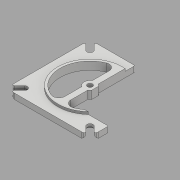
# Autodesk Inventor part: V4 In wall
Saved by Autodesk Inventor 2018 (Build 220112000, 112)
## iProperties
Created: 2020-01-08
Part Number: V4 In wall
Material: Generic
Document SubType Name: Modeling
Designer: user
Density: 1 g/cm^3
Appearance: Default
Author: user
Autodesk Inventor part; units mm, degrees
ref_plane "YZ Plane" through (0, 0, 0) normal (1, 0, 0) x (0, 1, 0)
ref_plane "XZ Plane" through (0, 0, 0) normal (0, 1, 0) x (-1, 0, 0)
ref_plane "XY Plane" through (0, 0, 0) normal (0, 0, 1) x (1, 0, 0)
sketch "Sketch1" plane through (0, 0, 0) normal (0, 0, 1) x (1, 0, 0)
  line L0 (-28.2, -35.2) -> (28.2, -35.2)
  line L1 (35.2, -28.2) -> (35.2, 28.2)
  line L2 (28.2, 35.2) -> (-28.2, 35.2)
  line L3 (-35.2, 28.2) -> (-35.2, -28.2)
  line L4 (-35.2, -35.2) -> (35.2, 35.2) construction
  line L5 (35.2, -35.2) -> (-35.2, 35.2) construction
  arc A0 (-28.2, 35.2) -> (-35.2, 28.2) centre (-28.2, 28.2) ccw
  arc A1 (35.2, 28.2) -> (28.2, 35.2) centre (28.2, 28.2) ccw
  arc A2 (-35.2, -28.2) -> (-28.2, -35.2) centre (-28.2, -28.2) ccw
  arc A3 (28.2, -35.2) -> (35.2, -28.2) centre (28.2, -28.2) ccw
  line L6 (-2.5, -24.8747) -> (2.5, -24.8747) construction
  line L7 (2.5, 24.8747) -> (-2.5, 24.8747) construction
  line L8 (-2.5, -24.8747) -> (2.5, 24.8747) construction
  line L9 (2.5, -24.8747) -> (-2.5, 24.8747) construction
  arc A4 (-9.375, 23.1756) -> (-9.375, -23.1756) centre (0, 0) ccw
  arc A5 (9.375, -23.1756) -> (9.375, 23.1756) centre (0, 0) ccw
  arc A6 (-2.5, 18.5405) -> (-9.375, 23.1756) centre (-7.5, 18.5405) ccw
  arc A7 (9.375, 23.1756) -> (2.5, 18.5405) centre (7.5, 18.5405) ccw
  arc A8 (-9.375, -23.1756) -> (-2.5, -18.5405) centre (-7.5, -18.5405) ccw
  arc A9 (2.5, -18.5405) -> (9.375, -23.1756) centre (7.5, -18.5405) ccw
  line L10 (2.5, 4.3301) -> (2.5, 18.5405)
  line L11 (-2.5, 18.5405) -> (-2.5, 4.3301)
  line L12 (-2.5, -4.3301) -> (-2.5, -18.5405)
  line L13 (2.5, -18.5405) -> (2.5, -4.3301)
  arc A10 (-2.5, 4.3301) -> (-2.5, -4.3301) centre (0, 0) ccw
  arc A11 (2.5, -4.3301) -> (2.5, 4.3301) centre (0, 0) ccw
  dimension "d0" = 70.4
  dimension "d1" = 7
  dimension "d3" = 5
  dimension "d4" = 25
  dimension "d5" = 5
  dimension "d7" = 5
  constraints: 28 end point, 28 point on circle, 20 tangent, 12 centre point, 10 point on line, 7 equal radius, 7 parallel, 4 midpoint, 4 perpendicular, 2 coincident, 2 horizontal
  measures "d0" distance of L4.end L5.end
  measures "d1" radius of A0
  measures "d3" distance of L7.end L7.start
  measures "d4" radius of A5
  measures "d5" radius of A6
  measures "d7" radius of A11
extrude "Extrusion1" add sketch "Sketch1" along normal blind 4.7
sketch "Sketch2" plane through (0, 0, 4.7) normal (0, 0, 1) x (1, 0, 0)
  circle A0 centre (0, 0) radius 27
  arc A1 (9.375, -23.1756) -> (9.375, 23.1756) centre (0, 0) ccw projected
  arc A2 (2.5, -18.5405) -> (9.375, -23.1756) centre (7.5, -18.5405) ccw projected
  line L0 (2.5, -18.5405) -> (2.5, -4.3301) projected
  arc A3 (2.5, -4.3301) -> (2.5, 4.3301) centre (0, 0) ccw projected
  line L1 (2.5, 4.3301) -> (2.5, 18.5405) projected
  arc A4 (9.375, 23.1756) -> (2.5, 18.5405) centre (7.5, 18.5405) ccw projected
  line L2 (-2.5, 18.5405) -> (-2.5, 4.3301) projected
  arc A5 (-2.5, 4.3301) -> (-2.5, -4.3301) centre (0, 0) ccw projected
  line L3 (-2.5, -4.3301) -> (-2.5, -18.5405) projected
  arc A6 (-9.375, -23.1756) -> (-2.5, -18.5405) centre (-7.5, -18.5405) ccw projected
  arc A7 (-9.375, 23.1756) -> (-9.375, -23.1756) centre (0, 0) ccw projected
  arc A8 (-2.5, 18.5405) -> (-9.375, 23.1756) centre (-7.5, 18.5405) ccw projected
  line L4 (28.2, 35.2) -> (-28.2, 35.2) projected
  arc A9 (-28.2, 35.2) -> (-35.2, 28.2) centre (-28.2, 28.2) ccw projected
  line L5 (-35.2, 28.2) -> (-35.2, -28.2) projected
  arc A10 (-35.2, -28.2) -> (-28.2, -35.2) centre (-28.2, -28.2) ccw projected
  line L6 (-28.2, -35.2) -> (28.2, -35.2) projected
  arc A11 (28.2, -35.2) -> (35.2, -28.2) centre (28.2, -28.2) ccw projected
  line L7 (35.2, -28.2) -> (35.2, 28.2) projected
  arc A12 (35.2, 28.2) -> (28.2, 35.2) centre (28.2, 28.2) ccw projected
  dimension "d10" = 54
  constraints: 1 centre point, 1 coincident
  measures "d10" diameter of A0
extrude "Extrusion2" add sketch "Sketch2" along normal blind 2 contours A0
sketch "Sketch3" plane through (0, 0, 0) normal (0, 0, -1) x (-1, 0, 0)
  line L0 (-27.5, -27.5) -> (27.5, -27.5) construction
  line L1 (27.5, -27.5) -> (27.5, 27.5) construction
  line L2 (27.5, 27.5) -> (-27.5, 27.5) construction
  line L3 (-27.5, 27.5) -> (-27.5, -27.5) construction
  line L4 (-27.5, -27.5) -> (27.5, 27.5) construction
  line L5 (27.5, -27.5) -> (-27.5, 27.5) construction
  line L6 (27.5, 27.5) -> (32.8233, 32.8233) construction
  line L7 (29.2678, 25.7322) -> (34.5911, 31.0555)
  line L8 (31.0555, 34.5911) -> (25.7322, 29.2678)
  arc A0 (25.7322, 29.2678) -> (29.2678, 25.7322) centre (27.5, 27.5) ccw
  arc A1 (34.5911, 31.0555) -> (31.0555, 34.5911) centre (32.8233, 32.8233) ccw
  arc A2 (35.2, 28.2) -> (28.2, 35.2) centre (28.2, 28.2) ccw construction
  line L9 (-25.7322, 29.2678) -> (-31.0555, 34.5911)
  arc A3 (-29.2678, 25.7322) -> (-25.7322, 29.2678) centre (-27.5, 27.5) ccw
  line L10 (-34.5911, 31.0555) -> (-29.2678, 25.7322)
  arc A4 (-31.0555, 34.5911) -> (-34.5911, 31.0555) centre (-32.8233, 32.8233) ccw
  line L11 (-29.2678, -25.7322) -> (-34.5911, -31.0555)
  arc A5 (-25.7322, -29.2678) -> (-29.2678, -25.7322) centre (-27.5, -27.5) ccw
  line L12 (-31.0555, -34.5911) -> (-25.7322, -29.2678)
  arc A6 (-34.5911, -31.0555) -> (-31.0555, -34.5911) centre (-32.8233, -32.8233) ccw
  line L13 (25.7322, -29.2678) -> (31.0555, -34.5911)
  arc A7 (29.2678, -25.7322) -> (25.7322, -29.2678) centre (27.5, -27.5) ccw
  line L14 (34.5911, -31.0555) -> (29.2678, -25.7322)
  arc A8 (31.0555, -34.5911) -> (34.5911, -31.0555) centre (32.8233, -32.8233) ccw
  point P0 (0, 0)
  point P1 (30.1617, 30.1617)
  dimension "d13" = 55
  dimension "d14" = 5
  dimension "d18" = 360
  constraints: 32 end point, 17 point on circle, 8 centre point, 4 tangent, 3 midpoint, 3 parallel, 2 perpendicular, 1 collinear, 1 horizontal, 41 other
  measures "d13" distance of L2.end L1.end
  measures "d14" distance between parallel lines of L7 L8
extrude "Extrusion3" cut sketch "Sketch3" against normal through all
chamfer "Chamfer1" distance 2.5 angle 45 12 edges at (28.3939, 31.9294, 0) (25.7322, 25.7322, 0) (31.9294, 28.3939, 0) (-28.3939, 31.9294, 0) (-25.7322, 25.7322, 0) (-31.9294, 28.3939, 0) (-25.7322, -25.7322, 0) (-31.9294, -28.3939, 0) (-28.3939, -31.9294, 0) (25.7322, -25.7322, 0) (28.3939, -31.9294, 0) (31.9294, -28.3939, 0)
fillet "Fillet1" radius 1 8 edges at (31.0555, 34.5911, 3.6) (34.5911, 31.0555, 3.6) (34.5911, -31.0555, 3.6) (31.0555, -34.5911, 3.6) (-31.0555, -34.5911, 3.6) (-34.5911, -31.0555, 3.6) (-34.5911, 31.0555, 3.6) (-31.0555, 34.5911, 3.6)
hole "Hole1" at (0, 0, 0) direction (0, 0, 1) diameter 4.2 end through all
sketch "Sketch4" plane through (0, 0, 0) normal (0, 0, -1) x (-1, 0, 0)
  line L0 (-35.2, 35.2) -> (-2.5, 35.2)
  line L1 (-2.5, 35.2) -> (-2.5, 4.3301)
  line L2 (-2.5, 4.3301) -> (-4.2, 4.3301)
  line L3 (-4.2, 4.3301) -> (-4.2, -19.8)
  line L4 (-4.2, -19.8) -> (-35.2, -19.8)
  line L5 (-35.2, 28.1289) -> (-35.2, -28.1289) construction
  line L6 (-35.2, 35.2) -> (-35.2, -19.8)
  line L7 (-2.5, 18.5405) -> (-2.5, 4.3301) projected
  line L8 (28.1289, 35.2) -> (-28.1289, 35.2) construction
  point P0 (0, 0)
  point P1 (2.5, 4.3301)
  dimension "d39" = 31
  dimension "d41" = 55
  constraints: 12 end point, 4 perpendicular, 3 collinear, 2 point on line, 1 horizontal
  measures "d39" distance between parallel lines of L6 L3
  measures "d41" distance of L0.start L4.end
extrude "Extrusion4" cut sketch "Sketch4" against normal through all
fillet "Fillet2" radius 1 3 edges at (35.2, -19.8, 2.35) (15.263, -19.8, 3.35) (2.5, 35.2, 2.35)
equation "\"Offset\" = 0.3"
body "Solid1"
